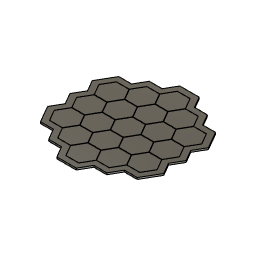
james-webb-v4 (Autodesk Fusion 360 design; units mm, degrees)
Autodesk Fusion 360 part; units mm, degrees
(part 1 of 5)
sketch "Sketch1" plane through (0, 0, 0) normal (0, 0, 1) x (1, 0, 0)
  line L0 (0, 0) -> (0, 112.8677) construction
  line L1 (-49.7965, 86.25) -> (-99.5929, 0)
  line L2 (-99.5929, 0) -> (-49.7965, -86.25)
  line L3 (-49.7965, -86.25) -> (49.7965, -86.25)
  line L4 (49.7965, -86.25) -> (99.5929, 0)
  line L5 (99.5929, 0) -> (49.7965, 86.25)
  line L6 (49.7965, 86.25) -> (-49.7965, 86.25)
  line L7 (0, 0) -> (74.6947, 43.125) construction
  line L8 (-252.4464, -88.25) -> (-352.0393, -88.25)
  line L9 (-352.0393, -88.25) -> (-401.8358, -174.5)
  line L10 (-401.8358, -174.5) -> (-352.0393, -260.75)
  line L11 (-352.0393, -260.75) -> (-252.4464, -260.75)
  line L12 (-252.4464, -260.75) -> (-202.6499, -174.5)
  line L13 (-202.6499, -174.5) -> (-252.4464, -88.25)
  line L14 (-101.325, -1) -> (-200.9179, -1)
  line L15 (-200.9179, -1) -> (-250.7144, -87.25)
  line L16 (-250.7144, -87.25) -> (-200.9179, -173.5)
  line L17 (-200.9179, -173.5) -> (-101.325, -173.5)
  line L18 (-101.325, -173.5) -> (-51.5285, -87.25)
  line L19 (-51.5285, -87.25) -> (-101.325, -1)
  line L20 (200.9179, 173.5) -> (101.325, 173.5)
  line L21 (101.325, 173.5) -> (51.5285, 87.25)
  line L22 (51.5285, 87.25) -> (101.325, 1)
  line L23 (101.325, 1) -> (200.9179, 1)
  line L24 (200.9179, 1) -> (250.7144, 87.25)
  line L25 (250.7144, 87.25) -> (200.9179, 173.5)
  line L26 (352.0393, 260.75) -> (252.4464, 260.75)
  line L27 (252.4464, 260.75) -> (202.6499, 174.5)
  line L28 (202.6499, 174.5) -> (252.4464, 88.25)
  line L29 (252.4464, 88.25) -> (352.0393, 88.25)
  line L30 (352.0393, 88.25) -> (401.8358, 174.5)
  line L31 (401.8358, 174.5) -> (352.0393, 260.75)
  line L32 (0, 0) -> (74.6947, -43.125) construction
  line L33 (-252.4464, 260.75) -> (-352.0393, 260.75)
  line L34 (-352.0393, 260.75) -> (-401.8358, 174.5)
  line L35 (-401.8358, 174.5) -> (-352.0393, 88.25)
  line L36 (-352.0393, 88.25) -> (-252.4464, 88.25)
  line L37 (-252.4464, 88.25) -> (-202.6499, 174.5)
  line L38 (-202.6499, 174.5) -> (-252.4464, 260.75)
  line L39 (-101.325, 173.5) -> (-200.9179, 173.5)
  line L40 (-200.9179, 173.5) -> (-250.7144, 87.25)
  line L41 (-250.7144, 87.25) -> (-200.9179, 1)
  line L42 (-200.9179, 1) -> (-101.325, 1)
  line L43 (-101.325, 1) -> (-51.5285, 87.25)
  line L44 (-51.5285, 87.25) -> (-101.325, 173.5)
  line L45 (200.9179, -1) -> (101.325, -1)
  line L46 (101.325, -1) -> (51.5285, -87.25)
  line L47 (51.5285, -87.25) -> (101.325, -173.5)
  line L48 (101.325, -173.5) -> (200.9179, -173.5)
  line L49 (200.9179, -173.5) -> (250.7144, -87.25)
  line L50 (250.7144, -87.25) -> (200.9179, -1)
  line L51 (352.0393, -88.25) -> (252.4464, -88.25)
  line L52 (252.4464, -88.25) -> (202.6499, -174.5)
  line L53 (202.6499, -174.5) -> (252.4464, -260.75)
  line L54 (252.4464, -260.75) -> (352.0393, -260.75)
  line L55 (352.0393, -260.75) -> (401.8358, -174.5)
  line L56 (401.8358, -174.5) -> (352.0393, -88.25)
  line L57 (99.5929, -349) -> (49.7965, -262.75)
  line L58 (49.7965, -262.75) -> (-49.7965, -262.75)
  line L59 (-49.7965, -262.75) -> (-99.5929, -349)
  line L60 (-99.5929, -349) -> (-49.7965, -435.25)
  line L61 (-49.7965, -435.25) -> (49.7965, -435.25)
  line L62 (49.7965, -435.25) -> (99.5929, -349)
  line L63 (99.5929, -174.5) -> (49.7965, -88.25)
  line L64 (49.7965, -88.25) -> (-49.7965, -88.25)
  line L65 (-49.7965, -88.25) -> (-99.5929, -174.5)
  line L66 (-99.5929, -174.5) -> (-49.7965, -260.75)
  line L67 (-49.7965, -260.75) -> (49.7965, -260.75)
  line L68 (49.7965, -260.75) -> (99.5929, -174.5)
  line L69 (99.5929, 174.5) -> (49.7965, 260.75)
  line L70 (49.7965, 260.75) -> (-49.7965, 260.75)
  line L71 (-49.7965, 260.75) -> (-99.5929, 174.5)
  line L72 (-99.5929, 174.5) -> (-49.7965, 88.25)
  line L73 (-49.7965, 88.25) -> (49.7965, 88.25)
  line L74 (49.7965, 88.25) -> (99.5929, 174.5)
  line L75 (99.5929, 349) -> (49.7965, 435.25)
  line L76 (49.7965, 435.25) -> (-49.7965, 435.25)
  line L77 (-49.7965, 435.25) -> (-99.5929, 349)
  line L78 (-99.5929, 349) -> (-49.7965, 262.75)
  line L79 (-49.7965, 262.75) -> (49.7965, 262.75)
  line L80 (49.7965, 262.75) -> (99.5929, 349)
  line L81 (-225.8161, 44.125) -> (74.6947, 217.625) construction
  line L82 (-200.9179, 348) -> (-101.325, 348)
  line L83 (-101.325, 348) -> (-51.5285, 261.75)
  line L84 (-51.5285, 261.75) -> (-101.325, 175.5)
  line L85 (-101.325, 175.5) -> (-200.9179, 175.5)
  line L86 (-200.9179, 175.5) -> (-250.7144, 261.75)
  line L87 (-250.7144, 261.75) -> (-200.9179, 348)
  line L88 (51.5285, 261.75) -> (101.325, 175.5)
  line L89 (101.325, 175.5) -> (200.9179, 175.5)
  line L90 (200.9179, 175.5) -> (250.7144, 261.75)
  line L91 (250.7144, 261.75) -> (200.9179, 348)
  line L92 (200.9179, 348) -> (101.325, 348)
  line L93 (101.325, 348) -> (51.5285, 261.75)
  line L94 (151.1214, 173.5) -> (151.1214, 1) construction
  line L95 (401.8358, 0) -> (352.0393, -86.25)
  line L96 (352.0393, -86.25) -> (252.4464, -86.25)
  line L97 (252.4464, -86.25) -> (202.6499, 0)
  line L98 (202.6499, 0) -> (252.4464, 86.25)
  line L99 (252.4464, 86.25) -> (352.0393, 86.25)
  line L100 (352.0393, 86.25) -> (401.8358, 0)
  line L101 (250.7144, -261.75) -> (200.9179, -175.5)
  line L102 (200.9179, -175.5) -> (101.325, -175.5)
  line L103 (101.325, -175.5) -> (51.5285, -261.75)
  line L104 (51.5285, -261.75) -> (101.325, -348)
  line L105 (101.325, -348) -> (200.9179, -348)
  line L106 (200.9179, -348) -> (250.7144, -261.75)
  line L107 (-151.1214, 173.5) -> (-151.1214, -173.5) construction
  line L108 (-401.8358, 0) -> (-352.0393, 86.25)
  line L109 (-352.0393, 86.25) -> (-252.4464, 86.25)
  line L110 (-252.4464, 86.25) -> (-202.6499, 0)
  line L111 (-202.6499, 0) -> (-252.4464, -86.25)
  line L112 (-252.4464, -86.25) -> (-352.0393, -86.25)
  line L113 (-352.0393, -86.25) -> (-401.8358, 0)
  line L114 (-101.325, -348) -> (-51.5285, -261.75)
  line L115 (-51.5285, -261.75) -> (-101.325, -175.5)
  line L116 (-101.325, -175.5) -> (-200.9179, -175.5)
  line L117 (-200.9179, -175.5) -> (-250.7144, -261.75)
  line L118 (-250.7144, -261.75) -> (-200.9179, -348)
  line L119 (-200.9179, -348) -> (-101.325, -348)
  line L120 (138.5641, 371.5) -> (75.7772, 480.25)
  line L121 (75.7772, 480.25) -> (-75.7772, 480.25)
  line L122 (-75.7772, 480.25) -> (-138.5641, 371.5)
  line L123 (289.6855, 284.25) -> (226.8987, 393)
  line L124 (226.8987, 393) -> (101.325, 393)
  line L125 (391.0105, 65.75) -> (453.7973, 174.5)
  line L126 (453.7973, 174.5) -> (378.0201, 305.75)
  line L127 (378.0201, 305.75) -> (252.4464, 305.75)
  line L128 (391.0105, 108.75) -> (453.7973, 0)
  line L129 (453.7973, 0) -> (391.0105, -108.75)
  line L130 (252.4464, -305.75) -> (378.0201, -305.75)
  line L131 (378.0201, -305.75) -> (453.7973, -174.5)
  line L132 (453.7973, -174.5) -> (391.0105, -65.75)
  line L133 (101.325, -393) -> (226.8987, -393)
  line L134 (226.8987, -393) -> (289.6855, -284.25)
  line L135 (-138.5641, -371.5) -> (-75.7772, -480.25)
  line L136 (-75.7772, -480.25) -> (75.7772, -480.25)
  line L137 (75.7772, -480.25) -> (138.5641, -371.5)
  line L138 (-289.6855, -284.25) -> (-226.8987, -393)
  line L139 (-226.8987, -393) -> (-101.325, -393)
  line L140 (-391.0105, -65.75) -> (-453.7973, -174.5)
  line L141 (-453.7973, -174.5) -> (-378.0201, -305.75)
  line L142 (-378.0201, -305.75) -> (-252.4464, -305.75)
  line L143 (-391.0105, -108.75) -> (-453.7973, 0)
  line L144 (-453.7973, 0) -> (-391.0105, 108.75)
  line L145 (-252.4464, 305.75) -> (-378.0201, 305.75)
  line L146 (-378.0201, 305.75) -> (-453.7973, 174.5)
  line L147 (-453.7973, 174.5) -> (-391.0105, 65.75)
  line L148 (-289.6855, 284.25) -> (-226.8987, 393)
  line L149 (-226.8987, 393) -> (-101.325, 393)
  dimension "d2" = 86.25
  dimension "d12" = 174.5
  dimension "d13" = 0
  dimension "d16" = 174.5
  dimension "d17" = 0
  dimension "d20" = 174.5
  dimension "d21" = 0
  dimension "d23" = 45
  dimension "d24" = 45
  dimension "d25" = 45
  dimension "d27" = 45
  dimension "d28" = 45
  dimension "d29" = 45
  dimension "d30" = 45
  dimension "d31" = 45
  dimension "d33" = 45
  constraint coincident L0.start L7.start
  constraint vertical L0
  constraint midpoint L5 L7.end
  constraint midpoint L4 L32.end
  constraint perpendicular L4 L32
  constraint midpoint L41 L81.start
  constraint midpoint L69 L81.end
  constraint perpendicular L69 L81
  constraint symmetric L1.start L81 L84.end
  constraint symmetric L1.end L81 L85.end
  constraint symmetric L2.end L81 L86.end
  constraint symmetric L3.end L81 L82.start
  constraint symmetric L4.end L81 L82.end
  constraint symmetric L5.end L81 L83.end
  constraint symmetric L0 L82.start L91.end
  constraint symmetric L0 L82.end L92.end
  constraint symmetric L0 L83.end L88.start
  constraint symmetric L0 L84.end L88.end
  constraint symmetric L0 L85.end L89.end
  constraint symmetric L0 L86.end L90.end
  constraint midpoint L20 L94.start
  constraint midpoint L23 L94.end
  constraint perpendicular L23 L94
  constraint symmetric L1.start L94 L99.end
  constraint symmetric L1.end L94 L95.start
  constraint symmetric L2.end L94 L95.end
  constraint symmetric L3.end L94 L96.end
  constraint symmetric L4.end L94 L97.end
  constraint symmetric L5.end L94 L98.end
  constraint symmetric L32 L95.start L105.end
  constraint symmetric L32 L95.end L101.start
  constraint symmetric L32 L96.end L101.end
  constraint symmetric L32 L97.end L102.end
  constraint symmetric L32 L98.end L103.end
  constraint symmetric L32 L99.end L104.end
  constraint midpoint L39 L107.start
  constraint midpoint L17 L107.end
  constraint perpendicular L17 L107
  constraint symmetric L1.start L107 L109.end
  constraint symmetric L1.end L107 L110.end
  constraint symmetric L2.end L107 L111.end
  constraint symmetric L3.end L107 L112.end
  constraint symmetric L4.end L107 L108.start
  constraint symmetric L5.end L107 L108.end
  constraint symmetric L7 L108.start L118.end
  constraint symmetric L7 L108.end L114.start
  constraint symmetric L7 L109.end L114.end
  constraint symmetric L7 L110.end L115.end
  constraint symmetric L7 L111.end L116.end
  constraint symmetric L7 L112.end L117.end
  measures "d2" distance of L0.start L6
extrude "Extrude1" add sketch "Sketch1" against normal blind 12.7 contours L1 L2 L3 L4 L5 L6 | L8 L9 L10 L11 L12 L13 | L14 L15 L16 L17 L18 L19 | L20 L21 L22 L23 L24 L25 | L26 L27 L28 L29 L30 L31 | L33 L34 L35 L36 L37 L38 | L39 L40 L41 L42 L43 L44 | L45 L46 L47 L48 L49 L50 | L51 L52 L53 L54 L55 L56 | L57 L58 L59 L60 L61 L62 | L63 L64 L65 L66 L67 L68 | L69 L70 L71 L72 L73 L74 | L75 L76 L77 L78 L79 L80 | L82 L83 L84 L85 L86 L87 | L88 L89 L90 L91 L92 L93 | L95 L96 L97 L98 L99 L100 | L101 L102 L103 L104 L105 L106 | L108 L109 L110 L111 L112 L113 | L114 L115 L116 L117 L118 L119 | L120 L121 L122 L123 L124 L125 L126 L127 L128 L129 L130 L131 L132 L133 L134 L135 L136 L137 L138 L139 L140 L141 L142 L143 L144 L145 L146 L147 L148 L149 makes body 1
extrude "Extrude2" cut sketch "Sketch1" against normal blind 1 contours L1 L2 L3 L4 L5 L6 | L8 L9 L10 L11 L12 L13 | L14 L15 L16 L17 L18 L19 | L20 L21 L22 L23 L24 L25 | L26 L27 L28 L29 L30 L31 | L33 L34 L35 L36 L37 L38 | L39 L40 L41 L42 L43 L44 | L45 L46 L47 L48 L49 L50 | L51 L52 L53 L54 L55 L56 | L57 L58 L59 L60 L61 L62 | L63 L64 L65 L66 L67 L68 | L69 L70 L71 L72 L73 L74 | L75 L76 L77 L78 L79 L80 | L82 L83 L84 L85 L86 L87 | L88 L89 L90 L91 L92 L93 | L95 L96 L97 L98 L99 L100 | L101 L102 L103 L104 L105 L106 | L108 L109 L110 L111 L112 L113 | L114 L115 L116 L117 L118 L119 bodies 1
sketch "Mounting Features" plane through (0, 0, 0) normal (0, 0, 1) x (1, 0, 0) in component "SpoilBoard"
  line L0 (0, 0) -> (1219.2, 0)
  line L1 (1219.2, 0) -> (1219.2, 2463.8)
  line L2 (0, 2463.8) -> (0, 0)
  circle A0 centre (609.6, 20) radius 17.145
  line L3 (616.5977, 25.08) -> (602.6023, 25.08)
  arc A1 (602.6023, 25.08) -> (602.6023, 14.92) centre (602.6023, 20) ccw
  line L4 (602.6023, 14.92) -> (616.5977, 14.92)
  arc A2 (616.5977, 14.92) -> (616.5977, 25.08) centre (616.5977, 20) ccw
  line L5 (616.5977, 20) -> (602.6023, 20) construction
  line L6 (609.6, 0) -> (609.6, 20)
  arc A3 (27.2923, 25.08) -> (27.2923, 14.92) centre (27.2923, 20) ccw
  circle A4 centre (34.29, 20) radius 17.145
  line L7 (41.2877, 20) -> (27.2923, 20) construction
  arc A5 (41.2877, 14.92) -> (41.2877, 25.08) centre (41.2877, 20) ccw
  line L8 (41.2877, 25.08) -> (27.2923, 25.08)
  line L9 (27.2923, 14.92) -> (41.2877, 14.92)
  arc A6 (314.9473, 25.08) -> (314.9473, 14.92) centre (314.9473, 20) ccw
  circle A7 centre (321.945, 20) radius 17.145
  line L10 (328.9427, 20) -> (314.9473, 20) construction
  arc A8 (328.9427, 14.92) -> (328.9427, 25.08) centre (328.9427, 20) ccw
  line L11 (328.9427, 25.08) -> (314.9473, 25.08)
  line L12 (314.9473, 14.92) -> (328.9427, 14.92)
  arc A9 (890.2573, 25.08) -> (890.2573, 14.92) centre (890.2573, 20) ccw
  circle A10 centre (897.255, 20) radius 17.145
  line L13 (904.2527, 20) -> (890.2573, 20) construction
  arc A11 (904.2527, 14.92) -> (904.2527, 25.08) centre (904.2527, 20) ccw
  line L14 (904.2527, 25.08) -> (890.2573, 25.08)
  line L15 (890.2573, 14.92) -> (904.2527, 14.92)
  arc A12 (1177.9123, 25.08) -> (1177.9123, 14.92) centre (1177.9123, 20) ccw
  circle A13 centre (1184.91, 20) radius 17.145
  line L16 (1191.9077, 20) -> (1177.9123, 20) construction
  arc A14 (1191.9077, 14.92) -> (1191.9077, 25.08) centre (1191.9077, 20) ccw
  line L17 (1191.9077, 25.08) -> (1177.9123, 25.08)
  line L18 (1177.9123, 14.92) -> (1191.9077, 14.92)
  line L19 (0, 2463.8) -> (1219.2, 2463.8)
  circle A15 centre (34.29, 420) radius 17.145
  line L20 (41.2877, 425.08) -> (27.2923, 425.08)
  arc A16 (41.2877, 414.92) -> (41.2877, 425.08) centre (41.2877, 420) ccw
  line L21 (27.2923, 414.92) -> (41.2877, 414.92)
  arc A17 (27.2923, 425.08) -> (27.2923, 414.92) centre (27.2923, 420) ccw
  line L22 (41.2877, 420) -> (27.2923, 420) construction
  circle A18 centre (321.945, 420) radius 17.145
  line L23 (328.9427, 425.08) -> (314.9473, 425.08)
  arc A19 (328.9427, 414.92) -> (328.9427, 425.08) centre (328.9427, 420) ccw
  line L24 (314.9473, 414.92) -> (328.9427, 414.92)
  arc A20 (314.9473, 425.08) -> (314.9473, 414.92) centre (314.9473, 420) ccw
  line L25 (328.9427, 420) -> (314.9473, 420) construction
  line L26 (616.5977, 425.08) -> (602.6023, 425.08)
  arc A21 (602.6023, 425.08) -> (602.6023, 414.92) centre (602.6023, 420) ccw
  line L27 (602.6023, 414.92) -> (616.5977, 414.92)
  arc A22 (616.5977, 414.92) -> (616.5977, 425.08) centre (616.5977, 420) ccw
  line L28 (616.5977, 420) -> (602.6023, 420) construction
  circle A23 centre (609.6, 420) radius 17.145
  circle A24 centre (897.255, 420) radius 17.145
  line L29 (904.2527, 425.08) -> (890.2573, 425.08)
  arc A25 (904.2527, 414.92) -> (904.2527, 425.08) centre (904.2527, 420) ccw
  line L30 (890.2573, 414.92) -> (904.2527, 414.92)
  arc A26 (890.2573, 425.08) -> (890.2573, 414.92) centre (890.2573, 420) ccw
  line L31 (904.2527, 420) -> (890.2573, 420) construction
  line L32 (1191.9077, 425.08) -> (1177.9123, 425.08)
  arc A27 (1191.9077, 414.92) -> (1191.9077, 425.08) centre (1191.9077, 420) ccw
  line L33 (1177.9123, 414.92) -> (1191.9077, 414.92)
  arc A28 (1177.9123, 425.08) -> (1177.9123, 414.92) centre (1177.9123, 420) ccw
  circle A29 centre (1184.91, 420) radius 17.145
  line L34 (1191.9077, 420) -> (1177.9123, 420) construction
  circle A30 centre (34.29, 820) radius 17.145
  line L35 (41.2877, 825.08) -> (27.2923, 825.08)
  arc A31 (41.2877, 814.92) -> (41.2877, 825.08) centre (41.2877, 820) ccw
  line L36 (27.2923, 814.92) -> (41.2877, 814.92)
  arc A32 (27.2923, 825.08) -> (27.2923, 814.92) centre (27.2923, 820) ccw
  line L37 (41.2877, 820) -> (27.2923, 820) construction
  circle A33 centre (321.945, 820) radius 17.145
  line L38 (328.9427, 825.08) -> (314.9473, 825.08)
  arc A34 (328.9427, 814.92) -> (328.9427, 825.08) centre (328.9427, 820) ccw
  line L39 (314.9473, 814.92) -> (328.9427, 814.92)
  arc A35 (314.9473, 825.08) -> (314.9473, 814.92) centre (314.9473, 820) ccw
  line L40 (328.9427, 820) -> (314.9473, 820) construction
  line L41 (616.5977, 825.08) -> (602.6023, 825.08)
  arc A36 (602.6023, 825.08) -> (602.6023, 814.92) centre (602.6023, 820) ccw
  line L42 (602.6023, 814.92) -> (616.5977, 814.92)
  arc A37 (616.5977, 814.92) -> (616.5977, 825.08) centre (616.5977, 820) ccw
  line L43 (616.5977, 820) -> (602.6023, 820) construction
  circle A38 centre (609.6, 820) radius 17.145
  circle A39 centre (897.255, 820) radius 17.145
  line L44 (904.2527, 825.08) -> (890.2573, 825.08)
  arc A40 (904.2527, 814.92) -> (904.2527, 825.08) centre (904.2527, 820) ccw
  line L45 (890.2573, 814.92) -> (904.2527, 814.92)
  arc A41 (890.2573, 825.08) -> (890.2573, 814.92) centre (890.2573, 820) ccw
  line L46 (904.2527, 820) -> (890.2573, 820) construction
  line L47 (1191.9077, 825.08) -> (1177.9123, 825.08)
  arc A42 (1191.9077, 814.92) -> (1191.9077, 825.08) centre (1191.9077, 820) ccw
  line L48 (1177.9123, 814.92) -> (1191.9077, 814.92)
  arc A43 (1177.9123, 825.08) -> (1177.9123, 814.92) centre (1177.9123, 820) ccw
  circle A44 centre (1184.91, 820) radius 17.145
  line L49 (1191.9077, 820) -> (1177.9123, 820) construction
  circle A45 centre (34.29, 1220) radius 17.145
  line L50 (41.2877, 1225.08) -> (27.2923, 1225.08)
  arc A46 (41.2877, 1214.92) -> (41.2877, 1225.08) centre (41.2877, 1220) ccw
  line L51 (27.2923, 1214.92) -> (41.2877, 1214.92)
  arc A47 (27.2923, 1225.08) -> (27.2923, 1214.92) centre (27.2923, 1220) ccw
  line L52 (41.2877, 1220) -> (27.2923, 1220) construction
  circle A48 centre (321.945, 1220) radius 17.145
  line L53 (328.9427, 1225.08) -> (314.9473, 1225.08)
  arc A49 (328.9427, 1214.92) -> (328.9427, 1225.08) centre (328.9427, 1220) ccw
  line L54 (314.9473, 1214.92) -> (328.9427, 1214.92)
  arc A50 (314.9473, 1225.08) -> (314.9473, 1214.92) centre (314.9473, 1220) ccw
  line L55 (328.9427, 1220) -> (314.9473, 1220) construction
  line L56 (616.5977, 1225.08) -> (602.6023, 1225.08)
  arc A51 (602.6023, 1225.08) -> (602.6023, 1214.92) centre (602.6023, 1220) ccw
  line L57 (602.6023, 1214.92) -> (616.5977, 1214.92)
  arc A52 (616.5977, 1214.92) -> (616.5977, 1225.08) centre (616.5977, 1220) ccw
  line L58 (616.5977, 1220) -> (602.6023, 1220) construction
  circle A53 centre (609.6, 1220) radius 17.145
  circle A54 centre (897.255, 1220) radius 17.145
  line L59 (904.2527, 1225.08) -> (890.2573, 1225.08)
  arc A55 (904.2527, 1214.92) -> (904.2527, 1225.08) centre (904.2527, 1220) ccw
  line L60 (890.2573, 1214.92) -> (904.2527, 1214.92)
  arc A56 (890.2573, 1225.08) -> (890.2573, 1214.92) centre (890.2573, 1220) ccw
  line L61 (904.2527, 1220) -> (890.2573, 1220) construction
  line L62 (1191.9077, 1225.08) -> (1177.9123, 1225.08)
  arc A57 (1191.9077, 1214.92) -> (1191.9077, 1225.08) centre (1191.9077, 1220) ccw
  line L63 (1177.9123, 1214.92) -> (1191.9077, 1214.92)
  arc A58 (1177.9123, 1225.08) -> (1177.9123, 1214.92) centre (1177.9123, 1220) ccw
  circle A59 centre (1184.91, 1220) radius 17.145
  line L64 (1191.9077, 1220) -> (1177.9123, 1220) construction
  circle A60 centre (34.29, 1620) radius 17.145
  line L65 (41.2877, 1625.08) -> (27.2923, 1625.08)
  arc A61 (41.2877, 1614.92) -> (41.2877, 1625.08) centre (41.2877, 1620) ccw
  line L66 (27.2923, 1614.92) -> (41.2877, 1614.92)
  arc A62 (27.2923, 1625.08) -> (27.2923, 1614.92) centre (27.2923, 1620) ccw
  line L67 (41.2877, 1620) -> (27.2923, 1620) construction
  circle A63 centre (321.945, 1620) radius 17.145
  line L68 (328.9427, 1625.08) -> (314.9473, 1625.08)
  arc A64 (328.9427, 1614.92) -> (328.9427, 1625.08) centre (328.9427, 1620) ccw
  line L69 (314.9473, 1614.92) -> (328.9427, 1614.92)
  arc A65 (314.9473, 1625.08) -> (314.9473, 1614.92) centre (314.9473, 1620) ccw
  line L70 (328.9427, 1620) -> (314.9473, 1620) construction
  line L71 (616.5977, 1625.08) -> (602.6023, 1625.08)
  arc A66 (602.6023, 1625.08) -> (602.6023, 1614.92) centre (602.6023, 1620) ccw
  line L72 (602.6023, 1614.92) -> (616.5977, 1614.92)
  arc A67 (616.5977, 1614.92) -> (616.5977, 1625.08) centre (616.5977, 1620) ccw
  line L73 (616.5977, 1620) -> (602.6023, 1620) construction
  circle A68 centre (609.6, 1620) radius 17.145
  circle A69 centre (897.255, 1620) radius 17.145
  line L74 (904.2527, 1625.08) -> (890.2573, 1625.08)
  arc A70 (904.2527, 1614.92) -> (904.2527, 1625.08) centre (904.2527, 1620) ccw
  line L75 (890.2573, 1614.92) -> (904.2527, 1614.92)
  arc A71 (890.2573, 1625.08) -> (890.2573, 1614.92) centre (890.2573, 1620) ccw
  line L76 (904.2527, 1620) -> (890.2573, 1620) construction
  line L77 (1191.9077, 1625.08) -> (1177.9123, 1625.08)
  arc A72 (1191.9077, 1614.92) -> (1191.9077, 1625.08) centre (1191.9077, 1620) ccw
  line L78 (1177.9123, 1614.92) -> (1191.9077, 1614.92)
  arc A73 (1177.9123, 1625.08) -> (1177.9123, 1614.92) centre (1177.9123, 1620) ccw
  circle A74 centre (1184.91, 1620) radius 17.145
  line L79 (1191.9077, 1620) -> (1177.9123, 1620) construction
  circle A75 centre (34.29, 2020) radius 17.145
  line L80 (41.2877, 2025.08) -> (27.2923, 2025.08)
  arc A76 (41.2877, 2014.92) -> (41.2877, 2025.08) centre (41.2877, 2020) ccw
  line L81 (27.2923, 2014.92) -> (41.2877, 2014.92)
  arc A77 (27.2923, 2025.08) -> (27.2923, 2014.92) centre (27.2923, 2020) ccw
  line L82 (41.2877, 2020) -> (27.2923, 2020) construction
  circle A78 centre (321.945, 2020) radius 17.145
  line L83 (328.9427, 2025.08) -> (314.9473, 2025.08)
  arc A79 (328.9427, 2014.92) -> (328.9427, 2025.08) centre (328.9427, 2020) ccw
  line L84 (314.9473, 2014.92) -> (328.9427, 2014.92)
  arc A80 (314.9473, 2025.08) -> (314.9473, 2014.92) centre (314.9473, 2020) ccw
  line L85 (328.9427, 2020) -> (314.9473, 2020) construction
  line L86 (616.5977, 2025.08) -> (602.6023, 2025.08)
  arc A81 (602.6023, 2025.08) -> (602.6023, 2014.92) centre (602.6023, 2020) ccw
  line L87 (602.6023, 2014.92) -> (616.5977, 2014.92)
  arc A82 (616.5977, 2014.92) -> (616.5977, 2025.08) centre (616.5977, 2020) ccw
  line L88 (616.5977, 2020) -> (602.6023, 2020) construction
  circle A83 centre (609.6, 2020) radius 17.145
  circle A84 centre (897.255, 2020) radius 17.145
  line L89 (904.2527, 2025.08) -> (890.2573, 2025.08)
  arc A85 (904.2527, 2014.92) -> (904.2527, 2025.08) centre (904.2527, 2020) ccw
  line L90 (890.2573, 2014.92) -> (904.2527, 2014.92)
  arc A86 (890.2573, 2025.08) -> (890.2573, 2014.92) centre (890.2573, 2020) ccw
  line L91 (904.2527, 2020) -> (890.2573, 2020) construction
  line L92 (1191.9077, 2025.08) -> (1177.9123, 2025.08)
  arc A87 (1191.9077, 2014.92) -> (1191.9077, 2025.08) centre (1191.9077, 2020) ccw
  line L93 (1177.9123, 2014.92) -> (1191.9077, 2014.92)
  arc A88 (1177.9123, 2025.08) -> (1177.9123, 2014.92) centre (1177.9123, 2020) ccw
  circle A89 centre (1184.91, 2020) radius 17.145
  line L94 (1191.9077, 2020) -> (1177.9123, 2020) construction
  circle A90 centre (34.29, 2420) radius 17.145
  line L95 (41.2877, 2425.08) -> (27.2923, 2425.08)
  arc A91 (41.2877, 2414.92) -> (41.2877, 2425.08) centre (41.2877, 2420) ccw
  line L96 (27.2923, 2414.92) -> (41.2877, 2414.92)
  arc A92 (27.2923, 2425.08) -> (27.2923, 2414.92) centre (27.2923, 2420) ccw
  line L97 (41.2877, 2420) -> (27.2923, 2420) construction
  circle A93 centre (321.945, 2420) radius 17.145
  line L98 (328.9427, 2425.08) -> (314.9473, 2425.08)
  arc A94 (328.9427, 2414.92) -> (328.9427, 2425.08) centre (328.9427, 2420) ccw
  line L99 (314.9473, 2414.92) -> (328.9427, 2414.92)
  arc A95 (314.9473, 2425.08) -> (314.9473, 2414.92) centre (314.9473, 2420) ccw
  line L100 (328.9427, 2420) -> (314.9473, 2420) construction
  line L101 (616.5977, 2425.08) -> (602.6023, 2425.08)
  arc A96 (602.6023, 2425.08) -> (602.6023, 2414.92) centre (602.6023, 2420) ccw
  line L102 (602.6023, 2414.92) -> (616.5977, 2414.92)
  arc A97 (616.5977, 2414.92) -> (616.5977, 2425.08) centre (616.5977, 2420) ccw
  line L103 (616.5977, 2420) -> (602.6023, 2420) construction
  circle A98 centre (609.6, 2420) radius 17.145
  circle A99 centre (897.255, 2420) radius 17.145
  line L104 (904.2527, 2425.08) -> (890.2573, 2425.08)
  arc A100 (904.2527, 2414.92) -> (904.2527, 2425.08) centre (904.2527, 2420) ccw
  line L105 (890.2573, 2414.92) -> (904.2527, 2414.92)
  arc A101 (890.2573, 2425.08) -> (890.2573, 2414.92) centre (890.2573, 2420) ccw
  line L106 (904.2527, 2420) -> (890.2573, 2420) construction
  line L107 (1191.9077, 2425.08) -> (1177.9123, 2425.08)
  arc A102 (1191.9077, 2414.92) -> (1191.9077, 2425.08) centre (1191.9077, 2420) ccw
  line L108 (1177.9123, 2414.92) -> (1191.9077, 2414.92)
  arc A103 (1177.9123, 2425.08) -> (1177.9123, 2414.92) centre (1177.9123, 2420) ccw
  circle A104 centre (1184.91, 2420) radius 17.145
  line L109 (1191.9077, 2420) -> (1177.9123, 2420) construction
  point P0 (609.6, 20)
  point P1 (34.29, 20)
  point P2 (34.29, 20)
  point P3 (321.945, 20)
  point P4 (321.945, 20)
  point P5 (897.255, 20)
  point P6 (897.255, 20)
  point P7 (1184.91, 20)
  point P8 (1184.91, 20)
  point P9 (34.29, 420)
  point P10 (34.29, 820)
  point P11 (34.29, 1220)
  point P12 (34.29, 1620)
  point P13 (34.29, 2020)
  point P14 (34.29, 2420)
  dimension "d1" = 1219.2
  dimension "d2_1" = 2463.8
  dimension "d12_1" = 34.29
  dimension "d14_1" = 13.9954
  dimension "d15_1" = 5.08
  dimension "d29_1" = 20
  dimension "d87" = 575.31
  dimension "d88" = 2800
  dimension "d101" = 0
  dimension "d102" = 400
  constraint horizontal L0
  constraint vertical L1
  constraint vertical L2
  constraint coincident L0.start L2.end
  constraint tangent L3 A1
  constraint tangent A1 L4
  constraint parallel L3 L4
  constraint tangent L4 A2
  constraint tangent L3 A2
  constraint horizontal L5
  constraint midpoint L5 P0
  constraint coincident P0 A0.centre
  constraint midpoint L0 L6.start
  constraint perpendicular L0 L6
  constraint perpendicular L1 L19
  measures "d1" distance of L0.start L0.end
  measures "d2_1" distance of L0.start L2.start
  measures "d12_1" diameter of A0
  measures "d14_1" distance of A2.centre A1.centre
  measures "d15_1" radius of A2
  measures "d29_1" distance of L6.start P0
sketch "Dog Hole Grid" plane through (0, 0, 0) normal (0, 0, 1) x (1, 0, 0) in component "SpoilBoard"
  line L0 (0, 0) -> (1219.2, 0)
  line L1 (1219.2, 0) -> (1219.2, 2463.8)
  line L2 (1219.2, 2463.8) -> (0, 2463.8)
  line L3 (0, 2463.8) -> (0, 0)
  circle A0 centre (609.6, 62.8625) radius 9.525
  line L4 (0, 0) -> (1219.2, 0)
  line L5 (609.6, 0) -> (609.6, 62.8625)
  circle A1 centre (19.05, 62.8625) radius 9.525
  circle A2 centre (166.6875, 62.8625) radius 9.525
  circle A3 centre (314.325, 62.8625) radius 9.525
  circle A4 centre (461.9625, 62.8625) radius 9.525
  circle A5 centre (757.2375, 62.8625) radius 9.525
  circle A6 centre (904.875, 62.8625) radius 9.525
  circle A7 centre (1052.5125, 62.8625) radius 9.525
  circle A8 centre (1200.15, 62.8625) radius 9.525
  circle A9 centre (19.05, 170.0031) radius 9.525
  circle A10 centre (166.6875, 170.0031) radius 9.525
  circle A11 centre (314.325, 170.0031) radius 9.525
  circle A12 centre (461.9625, 170.0031) radius 9.525
  circle A13 centre (609.6, 170.0031) radius 9.525
  circle A14 centre (757.2375, 170.0031) radius 9.525
  circle A15 centre (904.875, 170.0031) radius 9.525
  circle A16 centre (1052.5125, 170.0031) radius 9.525
  circle A17 centre (1200.15, 170.0031) radius 9.525
  circle A18 centre (19.05, 277.1438) radius 9.525
  circle A19 centre (166.6875, 277.1438) radius 9.525
  circle A20 centre (314.325, 277.1438) radius 9.525
  circle A21 centre (461.9625, 277.1438) radius 9.525
  circle A22 centre (609.6, 277.1438) radius 9.525
  circle A23 centre (757.2375, 277.1438) radius 9.525
  circle A24 centre (904.875, 277.1438) radius 9.525
  circle A25 centre (1052.5125, 277.1438) radius 9.525
  circle A26 centre (1200.15, 277.1438) radius 9.525
  circle A27 centre (19.05, 384.2844) radius 9.525
  circle A28 centre (166.6875, 384.2844) radius 9.525
  circle A29 centre (314.325, 384.2844) radius 9.525
  circle A30 centre (461.9625, 384.2844) radius 9.525
  circle A31 centre (609.6, 384.2844) radius 9.525
  circle A32 centre (757.2375, 384.2844) radius 9.525
  circle A33 centre (904.875, 384.2844) radius 9.525
  circle A34 centre (1052.5125, 384.2844) radius 9.525
  circle A35 centre (1200.15, 384.2844) radius 9.525
  circle A36 centre (757.2375, 462.8625) radius 9.525
  circle A37 centre (609.6, 570.0031) radius 9.525
  circle A38 centre (461.9625, 462.8625) radius 9.525
  circle A39 centre (314.325, 462.8625) radius 9.525
  circle A40 centre (314.325, 570.0031) radius 9.525
  circle A41 centre (19.05, 784.2844) radius 9.525
  circle A42 centre (166.6875, 784.2844) radius 9.525
  circle A43 centre (314.325, 784.2844) radius 9.525
  circle A44 centre (461.9625, 784.2844) radius 9.525
  circle A45 centre (461.9625, 570.0031) radius 9.525
  circle A46 centre (314.325, 677.1437) radius 9.525
  circle A47 centre (461.9625, 677.1437) radius 9.525
  circle A48 centre (19.05, 570.0031) radius 9.525
  circle A49 centre (166.6875, 462.8625) radius 9.525
  circle A50 centre (166.6875, 570.0031) radius 9.525
  circle A51 centre (19.05, 462.8625) radius 9.525
  circle A52 centre (19.05, 677.1437) radius 9.525
  circle A53 centre (166.6875, 677.1437) radius 9.525
  circle A54 centre (609.6, 784.2844) radius 9.525
  circle A55 centre (757.2375, 784.2844) radius 9.525
  circle A56 centre (904.875, 784.2844) radius 9.525
  circle A57 centre (904.875, 462.8625) radius 9.525
  circle A58 centre (609.6, 677.1437) radius 9.525
  circle A59 centre (757.2375, 677.1437) radius 9.525
  circle A60 centre (904.875, 677.1437) radius 9.525
  circle A61 centre (1052.5125, 784.2844) radius 9.525
  circle A62 centre (1200.15, 784.2844) radius 9.525
  circle A63 centre (1052.5125, 462.8625) radius 9.525
  circle A64 centre (1200.15, 462.8625) radius 9.525
  circle A65 centre (1052.5125, 570.0031) radius 9.525
  circle A66 centre (1200.15, 570.0031) radius 9.525
  circle A67 centre (1200.15, 677.1437) radius 9.525
  circle A68 centre (1052.5125, 677.1437) radius 9.525
  circle A69 centre (609.6, 462.8625) radius 9.525
  circle A70 centre (757.2375, 570.0031) radius 9.525
  circle A71 centre (904.875, 570.0031) radius 9.525
  circle A72 centre (757.2375, 862.8625) radius 9.525
  circle A73 centre (609.6, 970.0031) radius 9.525
  circle A74 centre (461.9625, 862.8625) radius 9.525
  circle A75 centre (314.325, 862.8625) radius 9.525
  circle A76 centre (314.325, 970.0031) radius 9.525
  circle A77 centre (19.05, 1184.2844) radius 9.525
  circle A78 centre (166.6875, 1184.2844) radius 9.525
  circle A79 centre (314.325, 1184.2844) radius 9.525
  circle A80 centre (461.9625, 1184.2844) radius 9.525
  circle A81 centre (461.9625, 970.0031) radius 9.525
  circle A82 centre (314.325, 1077.1437) radius 9.525
  circle A83 centre (461.9625, 1077.1437) radius 9.525
  circle A84 centre (19.05, 970.0031) radius 9.525
  circle A85 centre (166.6875, 862.8625) radius 9.525
  circle A86 centre (166.6875, 970.0031) radius 9.525
  circle A87 centre (19.05, 862.8625) radius 9.525
  circle A88 centre (19.05, 1077.1437) radius 9.525
  circle A89 centre (166.6875, 1077.1437) radius 9.525
  circle A90 centre (609.6, 1184.2844) radius 9.525
  circle A91 centre (757.2375, 1184.2844) radius 9.525
  circle A92 centre (904.875, 1184.2844) radius 9.525
  circle A93 centre (904.875, 862.8625) radius 9.525
  circle A94 centre (609.6, 1077.1437) radius 9.525
  circle A95 centre (757.2375, 1077.1437) radius 9.525
  circle A96 centre (904.875, 1077.1437) radius 9.525
  circle A97 centre (1052.5125, 1184.2844) radius 9.525
  circle A98 centre (1200.15, 1184.2844) radius 9.525
  circle A99 centre (1052.5125, 862.8625) radius 9.525
  circle A100 centre (1200.15, 862.8625) radius 9.525
  circle A101 centre (1052.5125, 970.0031) radius 9.525
  circle A102 centre (1200.15, 970.0031) radius 9.525
  circle A103 centre (1200.15, 1077.1437) radius 9.525
  circle A104 centre (1052.5125, 1077.1437) radius 9.525
  circle A105 centre (609.6, 862.8625) radius 9.525
  circle A106 centre (757.2375, 970.0031) radius 9.525
  circle A107 centre (904.875, 970.0031) radius 9.525
  circle A108 centre (757.2375, 1262.8625) radius 9.525
  circle A109 centre (609.6, 1370.0031) radius 9.525
  circle A110 centre (461.9625, 1262.8625) radius 9.525
  circle A111 centre (314.325, 1262.8625) radius 9.525
  circle A112 centre (314.325, 1370.0031) radius 9.525
  circle A113 centre (19.05, 1584.2844) radius 9.525
  circle A114 centre (166.6875, 1584.2844) radius 9.525
  circle A115 centre (314.325, 1584.2844) radius 9.525
  circle A116 centre (461.9625, 1584.2844) radius 9.525
  circle A117 centre (461.9625, 1370.0031) radius 9.525
  circle A118 centre (314.325, 1477.1438) radius 9.525
  circle A119 centre (461.9625, 1477.1438) radius 9.525
  circle A120 centre (19.05, 1370.0031) radius 9.525
  circle A121 centre (166.6875, 1262.8625) radius 9.525
  circle A122 centre (166.6875, 1370.0031) radius 9.525
  circle A123 centre (19.05, 1262.8625) radius 9.525
  circle A124 centre (19.05, 1477.1438) radius 9.525
  circle A125 centre (166.6875, 1477.1438) radius 9.525
  circle A126 centre (609.6, 1584.2844) radius 9.525
  circle A127 centre (757.2375, 1584.2844) radius 9.525
  circle A128 centre (904.875, 1584.2844) radius 9.525
  circle A129 centre (904.875, 1262.8625) radius 9.525
  circle A130 centre (609.6, 1477.1438) radius 9.525
  circle A131 centre (757.2375, 1477.1438) radius 9.525
  circle A132 centre (904.875, 1477.1438) radius 9.525
  circle A133 centre (1052.5125, 1584.2844) radius 9.525
  circle A134 centre (1200.15, 1584.2844) radius 9.525
  circle A135 centre (1052.5125, 1262.8625) radius 9.525
  circle A136 centre (1200.15, 1262.8625) radius 9.525
  circle A137 centre (1052.5125, 1370.0031) radius 9.525
  circle A138 centre (1200.15, 1370.0031) radius 9.525
  circle A139 centre (1200.15, 1477.1438) radius 9.525
  circle A140 centre (1052.5125, 1477.1438) radius 9.525
  circle A141 centre (609.6, 1262.8625) radius 9.525
  circle A142 centre (757.2375, 1370.0031) radius 9.525
  circle A143 centre (904.875, 1370.0031) radius 9.525
  circle A144 centre (757.2375, 1662.8625) radius 9.525
  circle A145 centre (609.6, 1770.0031) radius 9.525
  circle A146 centre (461.9625, 1662.8625) radius 9.525
  circle A147 centre (314.325, 1662.8625) radius 9.525
  circle A148 centre (314.325, 1770.0031) radius 9.525
  circle A149 centre (19.05, 1984.2844) radius 9.525
  circle A150 centre (166.6875, 1984.2844) radius 9.525
  circle A151 centre (314.325, 1984.2844) radius 9.525
  circle A152 centre (461.9625, 1984.2844) radius 9.525
  circle A153 centre (461.9625, 1770.0031) radius 9.525
  circle A154 centre (314.325, 1877.1438) radius 9.525
  circle A155 centre (461.9625, 1877.1438) radius 9.525
  circle A156 centre (19.05, 1770.0031) radius 9.525
  circle A157 centre (166.6875, 1662.8625) radius 9.525
  circle A158 centre (166.6875, 1770.0031) radius 9.525
  circle A159 centre (19.05, 1662.8625) radius 9.525
  circle A160 centre (19.05, 1877.1438) radius 9.525
  circle A161 centre (166.6875, 1877.1438) radius 9.525
  circle A162 centre (609.6, 1984.2844) radius 9.525
  circle A163 centre (757.2375, 1984.2844) radius 9.525
  circle A164 centre (904.875, 1984.2844) radius 9.525
  circle A165 centre (904.875, 1662.8625) radius 9.525
  circle A166 centre (609.6, 1877.1438) radius 9.525
  circle A167 centre (757.2375, 1877.1438) radius 9.525
  circle A168 centre (904.875, 1877.1438) radius 9.525
  circle A169 centre (1052.5125, 1984.2844) radius 9.525
  circle A170 centre (1200.15, 1984.2844) radius 9.525
  circle A171 centre (1052.5125, 1662.8625) radius 9.525
  circle A172 centre (1200.15, 1662.8625) radius 9.525
  circle A173 centre (1052.5125, 1770.0031) radius 9.525
  circle A174 centre (1200.15, 1770.0031) radius 9.525
  circle A175 centre (1200.15, 1877.1438) radius 9.525
  circle A176 centre (1052.5125, 1877.1438) radius 9.525
  circle A177 centre (609.6, 1662.8625) radius 9.525
  circle A178 centre (757.2375, 1770.0031) radius 9.525
  circle A179 centre (904.875, 1770.0031) radius 9.525
  circle A180 centre (757.2375, 2062.8625) radius 9.525
  circle A181 centre (609.6, 2170.0031) radius 9.525
  circle A182 centre (461.9625, 2062.8625) radius 9.525
  circle A183 centre (314.325, 2062.8625) radius 9.525
  circle A184 centre (314.325, 2170.0031) radius 9.525
  circle A185 centre (19.05, 2384.2844) radius 9.525
  circle A186 centre (166.6875, 2384.2844) radius 9.525
  circle A187 centre (314.325, 2384.2844) radius 9.525
  circle A188 centre (461.9625, 2384.2844) radius 9.525
  circle A189 centre (461.9625, 2170.0031) radius 9.525
  circle A190 centre (314.325, 2277.1438) radius 9.525
  circle A191 centre (461.9625, 2277.1438) radius 9.525
  circle A192 centre (19.05, 2170.0031) radius 9.525
  circle A193 centre (166.6875, 2062.8625) radius 9.525
  circle A194 centre (166.6875, 2170.0031) radius 9.525
  circle A195 centre (19.05, 2062.8625) radius 9.525
  circle A196 centre (19.05, 2277.1438) radius 9.525
  circle A197 centre (166.6875, 2277.1438) radius 9.525
  circle A198 centre (609.6, 2384.2844) radius 9.525
  circle A199 centre (757.2375, 2384.2844) radius 9.525
  circle A200 centre (904.875, 2384.2844) radius 9.525
  circle A201 centre (904.875, 2062.8625) radius 9.525
  circle A202 centre (609.6, 2277.1438) radius 9.525
  circle A203 centre (757.2375, 2277.1438) radius 9.525
  circle A204 centre (904.875, 2277.1438) radius 9.525
  circle A205 centre (1052.5125, 2384.2844) radius 9.525
  circle A206 centre (1200.15, 2384.2844) radius 9.525
  circle A207 centre (1052.5125, 2062.8625) radius 9.525
  circle A208 centre (1200.15, 2062.8625) radius 9.525
  circle A209 centre (1052.5125, 2170.0031) radius 9.525
  circle A210 centre (1200.15, 2170.0031) radius 9.525
  circle A211 centre (1200.15, 2277.1438) radius 9.525
  circle A212 centre (1052.5125, 2277.1438) radius 9.525
  circle A213 centre (609.6, 2062.8625) radius 9.525
  circle A214 centre (757.2375, 2170.0031) radius 9.525
  circle A215 centre (904.875, 2170.0031) radius 9.525
  point P0 (609.6, 462.8625)
  point P1 (609.6, 862.8625)
  point P2 (609.6, 1262.8625)
  point P3 (609.6, 1662.8625)
  point P4 (609.6, 2062.8625)
  dimension "d24_1" = 1219.2
  dimension "d25_1" = 2463.8
  dimension "d27_1" = 19.05
  dimension "d30_1" = 62.8625
  dimension "d36_1" = 0
  dimension "d37_1" = 0
  dimension "d40" = 0
  dimension "d41" = 0
  dimension "d44" = 590.55
  dimension "d45" = 321.4219
  dimension "d50" = 0
  dimension "d51" = 2000
  constraint horizontal L0
  constraint vertical L1
  constraint horizontal L2
  constraint vertical L3
  constraint coincident L0.start L3.end
  constraint midpoint L0 L5.start
  constraint perpendicular L0 L5
  constraint coincident A0.centre L5.end
  measures "d24_1" distance of L0.start L0.end
  measures "d25_1" distance of L0.start L2.end
  measures "d27_1" diameter of A0
  measures "d30_1" distance of L5.start A0.centre